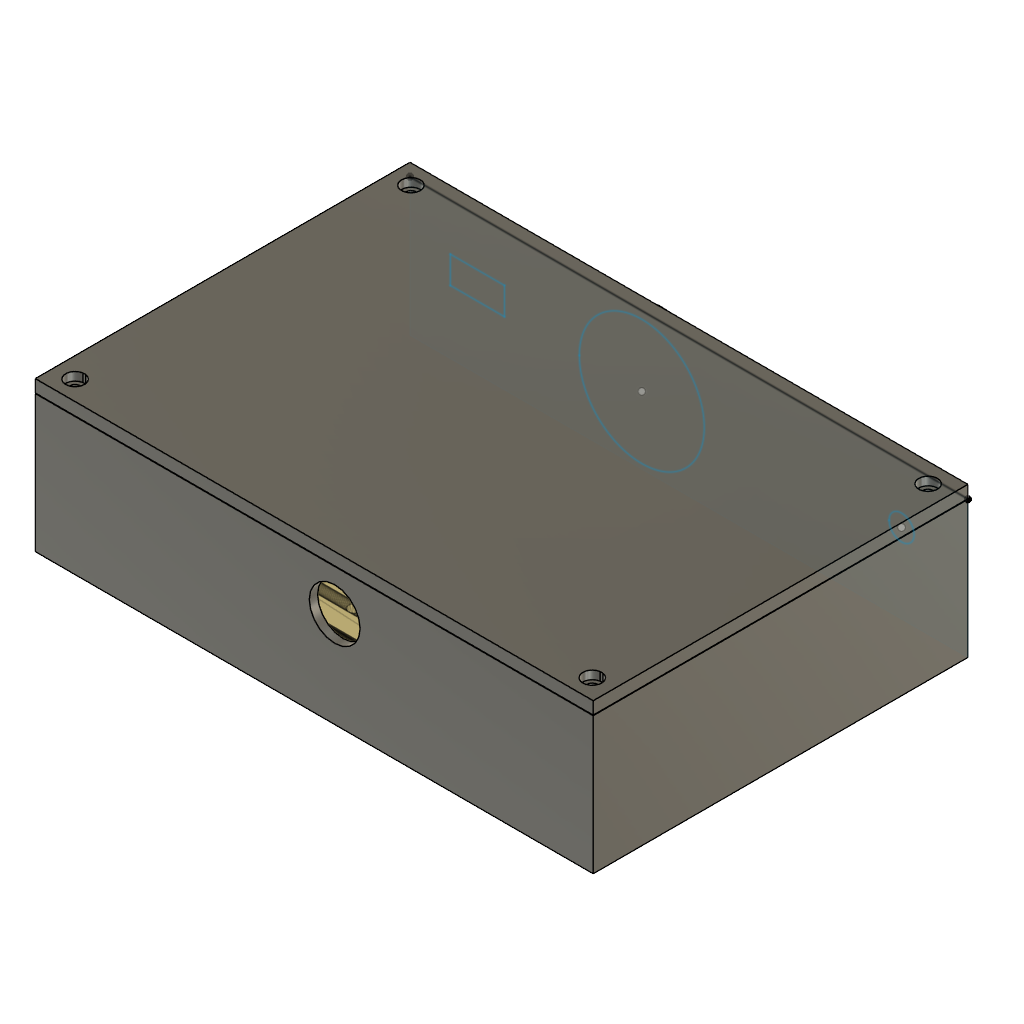
TerraVisionEnclosure (Autodesk Fusion 360 design; units mm, degrees)
part number: 2026-09-30-11-54-39-312
Autodesk Fusion 360 part; units mm, degrees
note: some values were not read from the file. Chosen so that the rebuilt part matches the saved one: which bodies a step acts on.
other "Elemento de malla base1"
other "Modificar1"
other "Modificar2"
other "Modificar3"
other "Modificar4"
other "Modificar5"
other "Modificar6"
other "Escala1"
other "Escala2"
other "Modificar7"
other "Modificar8"
other "Escala3"
sketch "Boceto3" plane through (0, 0, 0) normal (0, 0, 1) x (1, 0, 0)
  line L0 (-37.6392, 3.7951) -> (92.3608, 3.7951)
  line L1 (92.3608, 3.7951) -> (92.3608, 89.7951)
  line L2 (92.3608, 89.7951) -> (-37.6392, 89.7951)
  line L3 (-37.6392, 89.7951) -> (-37.6392, 3.7951)
  line L4 (92.1467, 91.7951) -> (-3.8533, 91.7951)
  line L5 (-3.8533, 1.7951) -> (92.1467, 1.7951)
  line L6 (94.3608, 1.7951) -> (94.3608, 91.7951)
  line L7 (94.3608, 91.7951) -> (-39.6392, 91.7951)
  line L8 (-39.6392, 91.7951) -> (-39.6392, 1.7951)
  line L9 (-39.6392, 1.7951) -> (94.3608, 1.7951)
  dimension "d25" = 130
  dimension "d26" = 86
  dimension "d27" = 2
  dimension "d28" = 2
  dimension "d29" = 2
  constraint horizontal L0
  constraint vertical L1
  constraint horizontal L2
  constraint vertical L3
  measures "d25" distance of L0.start L0.end
  measures "d26" distance of L0.end L1.end
extrude "Extruir1" add sketch "Boceto3" along normal blind 22 makes body 1
extrude "Extruir2" add 1 faces at (16.9561, 3.1284, 0) along direction (0, 0, -1) blind 2 on bodies 1 bodies 1
sketch "Boceto4" plane through (0, 0, -2) normal (0, 0, -1) x (1, 0, 0)
  line L0 (-37.6392, -89.7951) -> (-37.6392, -3.7951)
  line L1 (-37.6392, -3.7951) -> (92.3608, -3.7951)
  line L2 (92.3608, -3.7951) -> (92.3608, -89.7951)
  line L3 (92.3608, -89.7951) -> (-37.6392, -89.7951)
  line L4 (94.3608, -1.7951) -> (-39.6392, -1.7951)
  line L5 (-39.6392, -1.7951) -> (-39.6392, -91.7951)
  line L6 (-39.6392, -91.7951) -> (94.3608, -91.7951)
  line L7 (94.3608, -91.7951) -> (94.3608, -1.7951)
  line L8 (-39.6392, -1.7951) -> (94.3608, -1.7951)
  line L9 (94.3608, -1.7951) -> (94.3608, -91.7951)
  line L10 (94.3608, -91.7951) -> (-39.6392, -91.7951)
  line L11 (-39.6392, -91.7951) -> (-39.6392, -1.7951)
  line L12 (82.0002, -74) -> (87.2008, -74)
  line L13 (87.2008, -74) -> (87.2008, -77.8403)
  line L14 (87.2008, -77.8403) -> (82.0002, -77.8403)
  line L15 (82.0002, -77.8403) -> (82.0002, -74)
  line L16 (82.0002, -81.3917) -> (87.2008, -81.3917)
  line L17 (87.2008, -85.232) -> (82.0002, -85.232)
  line L18 (87.2008, -81.3917) -> (87.2008, -85.232)
  line L19 (82.0002, -85.232) -> (82.0002, -81.3917)
  line L20 (74.8756, -77.0003) -> (76.4831, -77.0003)
  line L21 (76.4831, -77.0003) -> (76.4831, -76.1982)
  line L22 (76.4831, -76.1982) -> (74.8756, -76.1982)
  line L23 (74.8756, -76.1982) -> (74.8756, -77.0003)
  line L24 (74.8706, -80.211) -> (76.4756, -80.211)
  line L25 (76.4756, -80.211) -> (76.4756, -81.0109)
  line L26 (76.4756, -81.0109) -> (74.8706, -81.0109)
  line L27 (74.8706, -81.0109) -> (74.8706, -80.211)
  line L28 (74.8675, -84.2259) -> (76.4935, -84.2259)
  line L29 (76.4935, -84.2259) -> (76.4935, -85.03)
  line L30 (76.4935, -85.03) -> (74.8675, -85.03)
  line L31 (74.8675, -85.03) -> (74.8675, -84.2259)
  line L32 (47.4882, -75.4522) -> (-31.5118, -75.4522)
  line L33 (-31.5118, -75.4522) -> (-31.5118, -37.9522)
  line L34 (-31.5118, -37.9522) -> (47.4882, -37.9522)
  line L35 (47.4882, -37.9522) -> (47.4882, -75.4522)
  circle A0 centre (77.0608, -61.7951) radius 6.5901
  line L36 (91.2608, -20.8951) -> (72.7608, -20.8951)
  line L37 (72.7608, -20.8951) -> (72.7608, -8.3951)
  line L38 (72.7608, -8.3951) -> (91.2608, -8.3951)
  line L39 (91.2608, -8.3951) -> (91.2608, -20.8951)
  circle A1 centre (51.0882, -73.0611) radius 2.25
  line L40 (7.9882, -33.9133) -> (7.9882, -79.4911) construction
  line L41 (51.6834, -56.7022) -> (-35.707, -56.7022) construction
  circle A2 centre (-35.1118, -73.0611) radius 2.25
  circle A3 centre (51.0882, -40.3432) radius 2.25
  circle A4 centre (-35.1118, -40.3432) radius 2.25
  circle A5 centre (3.5125, -87.4511) radius 1.5
  circle A6 centre (89.717, -87.3038) radius 1.5
  circle A7 centre (4.2711, -6.0742) radius 1.5
  circle A8 centre (89.46, -6.47) radius 1.5
  circle A9 centre (89.717, -87.3038) radius 1
  circle A10 centre (3.5125, -87.4511) radius 1
  circle A11 centre (4.2711, -6.0742) radius 1
  circle A12 centre (89.46, -6.47) radius 1
  point P0 (7.9882, -56.7022)
  point P1 (7.9882, -56.7022)
  dimension "d34" = 79
  dimension "d35" = 37.5
  dimension "d36" = 15.3
  dimension "d45" = 5.16
  dimension "d46" = 5.16
  dimension "d47" = 18.5
  dimension "d48" = 12.5
  dimension "d49" = 4.6
  dimension "d50" = 1.1
  dimension "d51" = 58
  dimension "d52" = 3.6
  dimension "d54" = 4.5
  dimension "d55" = 39.5
  dimension "d56" = 18.75
  dimension "d57" = 3
  dimension "d84" = -0.5
  dimension "d85" = -0.5
  dimension "d86" = -0.5
  dimension "d87" = -0.5
  constraint horizontal L8
  constraint vertical L9
  constraint horizontal L10
  constraint vertical L11
  constraint coincident L6.end L7.start
  constraint coincident L4.end L5.start
  constraint horizontal L12
  constraint vertical L13
  constraint horizontal L14
  constraint vertical L15
  constraint horizontal L16
  constraint vertical L18
  constraint horizontal L17
  constraint vertical L19
  constraint equal L12 L16
  constraint equal L15 L19
  constraint horizontal L20
  constraint vertical L21
  constraint horizontal L22
  constraint vertical L23
  constraint horizontal L24
  constraint vertical L25
  constraint horizontal L26
  constraint vertical L27
  constraint horizontal L28
  constraint vertical L29
  constraint horizontal L30
  constraint vertical L31
  constraint horizontal L32
  constraint vertical L33
  constraint horizontal L34
  constraint vertical L35
  constraint horizontal L36
  constraint vertical L37
  constraint horizontal L38
  constraint vertical L39
  constraint midpoint L40 P1
  constraint perpendicular L32 L40
  constraint midpoint L41 P1
  constraint coincident P1 P0
  constraint perpendicular L33 L41
  constraint symmetric A1 L40 A2
  constraint symmetric A1 L41 A3
  constraint symmetric L41 A2 A4
  constraint equal A5 A6
  constraint equal A5 A7
  constraint equal A5 A8
  measures "d34" distance of L32.start L32.end
  measures "d35" distance of L32.end L33.end
  measures "d36" distance of L2 A0.centre
  measures "d45" distance of L2 L13.end
  measures "d46" distance of L2 L17.start
  measures "d47" distance of L36.start L36.end
  measures "d48" distance of L36.start L38.end
  measures "d49" distance of L1 L38.end
  measures "d50" distance of L2 L38.end
  measures "d51" distance of L1 A0.centre
  measures "d52" distance of L35 A1.centre
  measures "d54" diameter of A1
  measures "d55" distance of L35 P1
  measures "d56" distance of L32 P1
  measures "d57" diameter of A5
extrude "Extruir6" add sketch "Boceto4" along normal blind 2 separate body contours L0 L1 L2 L3 makes body 2
extrude "Extruir7" add 1 faces at (49.0275, 2.4617, -2) along direction (0, 0, -1) blind 2 on bodies 1 bodies 1 2
extrude "Extruir8" add sketch "Boceto4" against normal blind 10 separate body contours A6 | A9 makes body 3
extrude "Extruir9" add sketch "Boceto4" against normal blind 10 separate body contours A5 | A7 | A8 | A10 | A11 | A12 makes body 4 at (4.9221, 86.9381, 4.6667) makes body 5 at (5.7693, 6.149, 4.6667) makes body 6 at (90.9581, 6.5448, 4.6667)
extrude "Extruir10" add 1 faces at (49.0275, 2.4617, 22) along direction (0, 0, 1) blind 7 on bodies 1 bodies 1
sketch "Boceto5" plane through (0, 1.7951, 0) normal (0, -1, 0) x (1, 0, 0)
  line L0 (94.3608, -4) -> (94.3608, 29)
  line L1 (94.3608, 29) -> (-39.6392, 29)
  line L2 (-39.6392, 29) -> (-39.6392, -4)
  line L3 (-39.6392, -4) -> (94.3608, -4)
  circle A0 centre (32.2847, 19) radius 6.1
  dimension "d68" = 12.2
  dimension "d69" = 33
  dimension "d70" = 23
  measures "d68" diameter of A0
  measures "d69" distance of L1 L3
  measures "d70" distance of L3 A0.centre
extrude "Extruir11" cut sketch "Boceto5" along normal blind -4 and the other way blind 0 contours A0 bodies 1
sketch "Boceto6" plane through (0, 91.7951, 0) normal (0, 1, 0) x (-1, 0, 0)
  line L0 (39.6392, -4) -> (39.6392, 29)
  line L1 (39.6392, 29) -> (-94.3608, 29)
  line L2 (-94.3608, 29) -> (-94.3608, -4)
  line L3 (-94.3608, -4) -> (39.6392, -4)
  line L4 (16.9478, 17.7095) -> (29.9478, 17.7095)
  line L5 (29.9478, 17.7095) -> (29.9478, 11.2095)
  line L6 (29.9478, 11.2095) -> (16.9478, 11.2095)
  line L7 (16.9478, 11.2095) -> (16.9478, 17.7095)
  circle A0 centre (-16.0339, 12.159) radius 15
  line L8 (39.6392, 29) -> (-94.3608, 29)
  line L9 (-94.3608, 29) -> (-94.3608, 28.9)
  line L10 (-94.3608, 28.9) -> (39.6392, 28.9)
  line L11 (39.6392, 28.9) -> (39.6392, 29)
  circle A1 centre (-78.4151, 15.0544) radius 3
  dimension "d75" = 6.5
  dimension "d76" = 13
  dimension "d77" = 30
  dimension "d135" = 0.1
  dimension "d141" = 6
  dimension "d146" = 33
  constraint horizontal L4
  constraint vertical L5
  constraint horizontal L6
  constraint vertical L7
  constraint horizontal L8
  constraint vertical L9
  constraint horizontal L10
  constraint vertical L11
  constraint coincident L2 L9.end
  constraint coincident L0.end L1.start
  measures "d75" distance of L4.end L5.end
  measures "d76" distance of L4.start L4.end
  measures "d77" diameter of A0
  measures "d135" distance of L0.end L10.end
  measures "d141" diameter of A1
  measures "d146" distance of L1.end L2.end
extrude "Extruir12" cut sketch "Boceto6" along normal blind -3 and the other way blind 0 contours L4 L5 L6 L7 bodies 1
extrude "Extruir13" add sketch "Boceto6" along normal blind 5 contours A0 bodies 1
extrude "Extruir14" cut sketch "Boceto4" against normal blind 10 contours A9 | A10 | A11 | A12 bodies 3 4 5 6
extrude "Extruir15" cut sketch "Boceto4" against normal blind 9 contours A5 | A6 | A7 | A8 bodies 3 4 5 6
sketch "Boceto7" plane through (0, 0, 29) normal (0, 0, 1) x (-1, 0, 0)
  line L0 (37.6392, -3.7951) -> (37.6392, -89.7951)
  line L1 (37.6392, -89.7951) -> (-92.3608, -89.7951)
  line L2 (-92.3608, -89.7951) -> (-92.3608, -3.7951)
  line L3 (-92.3608, -3.7951) -> (37.6392, -3.7951)
  line L4 (39.6392, -1.7951) -> (-94.3608, -1.7951)
  line L5 (-94.3608, -1.7951) -> (-94.3608, -91.7951)
  line L6 (-94.3608, -91.7951) -> (39.6392, -91.7951)
  line L7 (39.6392, -91.7951) -> (39.6392, -1.7951)
  line L8 (-89.1409, -8.6913) -> (-93.1409, -8.6913)
  line L9 (-93.1409, -8.6913) -> (-93.1409, -4.1913)
  line L10 (-93.1409, -4.1913) -> (-89.1409, -4.1913)
  line L11 (-87.1409, -6.1913) -> (-87.1409, -6.6913)
  arc A0 (-89.1409, -8.6913) -> (-87.1409, -6.6913) centre (-89.1409, -6.6913) ccw
  arc A1 (-87.1409, -6.1913) -> (-89.1409, -4.1913) centre (-89.1409, -6.1913) ccw
  circle A2 centre (-89.4569, -6.4674) radius 1.25
  line L12 (-94.3608, -1.7951) -> (-94.3608, -91.7951)
  line L13 (39.6392, -1.7951) -> (-94.3608, -1.7951)
  line L14 (65.6667, -46.7951) -> (-130, -46.7951) construction
  line L15 (-27.3608, -145) -> (-27.3608, 15) construction
  arc A3 (-87.1409, -86.8988) -> (-89.1409, -84.8988) centre (-89.1409, -86.8988) ccw
  line L16 (-89.1409, -84.8988) -> (-93.1409, -84.8988)
  line L17 (-93.1409, -84.8988) -> (-93.1409, -89.3988)
  line L18 (-93.1409, -89.3988) -> (-89.1409, -89.3988)
  arc A4 (-89.1409, -89.3988) -> (-87.1409, -87.3988) centre (-89.1409, -87.3988) ccw
  line L19 (-87.1409, -87.3988) -> (-87.1409, -86.8988)
  circle A5 centre (-89.4569, -87.1227) radius 1.25
  arc A6 (32.4192, -87.3988) -> (34.4192, -89.3988) centre (34.4192, -87.3988) ccw
  line L20 (38.4192, -89.3988) -> (34.4192, -89.3988)
  line L21 (38.4192, -84.8988) -> (38.4192, -89.3988)
  line L22 (34.4192, -84.8988) -> (38.4192, -84.8988)
  circle A7 centre (34.7353, -87.1227) radius 1.25
  arc A8 (34.4192, -84.8988) -> (32.4192, -86.8988) centre (34.4192, -86.8988) ccw
  line L23 (32.4192, -87.3988) -> (32.4192, -86.8988)
  line L24 (34.4192, -8.6913) -> (38.4192, -8.6913)
  line L25 (38.4192, -8.6913) -> (38.4192, -4.1913)
  line L26 (38.4192, -4.1913) -> (34.4192, -4.1913)
  arc A9 (34.4192, -4.1913) -> (32.4192, -6.1913) centre (34.4192, -6.1913) ccw
  arc A10 (32.4192, -6.6913) -> (34.4192, -8.6913) centre (34.4192, -6.6913) ccw
  line L27 (32.4192, -6.1913) -> (32.4192, -6.6913)
  circle A11 centre (34.7353, -6.4674) radius 1.25
  point P0 (-32.1667, -46.7951)
  point P1 (-27.3608, -65)
  dimension "d92" = 2
  dimension "d93" = 2
  dimension "d94" = 4.5
  dimension "d95" = 2.5
  dimension "d96" = 4
  dimension "d97" = 2
  dimension "d98" = 90
  dimension "d99" = 134
  dimension "d100" = 45
  dimension "d101" = 67
  constraint horizontal L8
  constraint vertical L9
  constraint horizontal L10
  constraint vertical L11
  constraint tangent L8 A0
  constraint tangent L11 A0
  constraint tangent L11 A1
  constraint tangent L10 A1
  constraint midpoint L14 P0
  constraint horizontal L14
  constraint midpoint L15 P1
  constraint perpendicular L13 L15
  constraint symmetric L8.end L14 L16.end
  constraint symmetric L9.end L14 L17.end
  constraint symmetric L8.start L14 A3.end
  constraint symmetric L11.end L14 A3.start
  constraint symmetric A0 L14 A3
  constraint symmetric L11.start L14 A4.end
  constraint symmetric L10.end L14 L18.end
  constraint symmetric A1 L14 A4
  constraint symmetric A2 L14 A5
  constraint symmetric L8.end L15 L24.end
  constraint symmetric L9.end L15 L25.end
  constraint symmetric L8.start L15 L24.start
  constraint symmetric L11.end L15 A10.start
  constraint symmetric A0 L15 A10
  constraint symmetric L11.start L15 A9.end
  constraint symmetric L10.end L15 L26.end
  constraint symmetric A1 L15 A9
  constraint symmetric A2 L15 A11
  constraint symmetric L15 A3.end L22.start
  constraint symmetric L15 A3.start A8.end
  constraint symmetric L15 A3 A8
  constraint symmetric L15 L16.end L21.start
  constraint symmetric L15 L17.end L20.start
  constraint symmetric L15 L18.end A6.end
  constraint symmetric L15 A4.end A6.start
  constraint symmetric L15 A4 A6
  constraint symmetric L15 A5 A7
  measures "d92" radius of A0
  measures "d93" radius of A1
  measures "d94" distance of L8.end L9.end
  measures "d95" diameter of A2
  measures "d96" distance of L8.end L8.start
  measures "d97" horizontal distance of L8.start L11.end
  measures "d98" distance of L4.end L5.end
  measures "d99" distance of L4.end L4.start
  measures "d100" distance of L13 L14
  measures "d101" distance of L12 L15
extrude "Extruir16" add sketch "Boceto7" against normal blind 2 contours L0 L24 L26 A9 A10 L27 | L2 L8 L10 L11 A0 A1 | L0 A6 L20 L22 A8 L23 | L2 A3 L16 L18 A4 L19 bodies 1
sketch "Boceto8" plane through (0, 0, 29) normal (0, 0, 1) x (-1, 0, 0)
  circle A0 centre (34.7353, -6.4674) radius 1.25
  circle A1 centre (34.7353, -87.1227) radius 1.25
  circle A2 centre (-89.4569, -6.4674) radius 1.25
  circle A3 centre (-89.4569, -87.1227) radius 1.25
  line L0 (37.6392, -3.7951) -> (37.6392, -4.1913)
  line L1 (37.6392, -4.1913) -> (34.4192, -4.1913)
  arc A4 (34.4192, -4.1913) -> (32.4192, -6.1913) centre (34.4192, -6.1913) ccw
  line L2 (32.4192, -6.1913) -> (32.4192, -6.6913)
  arc A5 (32.4192, -6.6913) -> (34.4192, -8.6913) centre (34.4192, -6.6913) ccw
  line L3 (34.4192, -8.6913) -> (37.6392, -8.6913)
  line L4 (37.6392, -8.6913) -> (37.6392, -84.8988)
  line L5 (37.6392, -84.8988) -> (34.4192, -84.8988)
  arc A6 (34.4192, -84.8988) -> (32.4192, -86.8988) centre (34.4192, -86.8988) ccw
  line L6 (32.4192, -86.8988) -> (32.4192, -87.3988)
  arc A7 (32.4192, -87.3988) -> (34.4192, -89.3988) centre (34.4192, -87.3988) ccw
  line L7 (34.4192, -89.3988) -> (37.6392, -89.3988)
  line L8 (37.6392, -89.3988) -> (37.6392, -89.7951)
  line L9 (37.6392, -89.7951) -> (-92.3608, -89.7951)
  line L10 (-92.3608, -89.7951) -> (-92.3608, -89.3988)
  line L11 (-92.3608, -89.3988) -> (-89.1409, -89.3988)
  arc A8 (-89.1409, -89.3988) -> (-87.1409, -87.3988) centre (-89.1409, -87.3988) ccw
  line L12 (-87.1409, -87.3988) -> (-87.1409, -86.8988)
  arc A9 (-87.1409, -86.8988) -> (-89.1409, -84.8988) centre (-89.1409, -86.8988) ccw
  line L13 (-89.1409, -84.8988) -> (-92.3608, -84.8988)
  line L14 (-92.3608, -84.8988) -> (-92.3608, -8.6913)
  line L15 (-92.3608, -8.6913) -> (-89.1409, -8.6913)
  arc A10 (-89.1409, -8.6913) -> (-87.1409, -6.6913) centre (-89.1409, -6.6913) ccw
  line L16 (-87.1409, -6.6913) -> (-87.1409, -6.1913)
  arc A11 (-87.1409, -6.1913) -> (-89.1409, -4.1913) centre (-89.1409, -6.1913) ccw
  line L17 (-89.1409, -4.1913) -> (-92.3608, -4.1913)
  line L18 (-92.3608, -4.1913) -> (-92.3608, -3.7951)
  line L19 (-92.3608, -3.7951) -> (37.6392, -3.7951)
  line L20 (39.6392, -1.7951) -> (-94.3608, -1.7951)
  line L21 (-94.3608, -1.7951) -> (-94.3608, -91.7951)
  line L22 (-94.3608, -91.7951) -> (39.6392, -91.7951)
  line L23 (39.6392, -91.7951) -> (39.6392, -1.7951)
  line L24 (39.6392, -1.7951) -> (-94.3608, -1.7951)
  line L25 (-94.3608, -1.7951) -> (-94.3608, -91.7951)
  line L26 (-94.3608, -91.7951) -> (39.6392, -91.7951)
  line L27 (39.6392, -91.7951) -> (39.6392, -1.7951)
  circle A12 centre (34.7353, -87.1227) radius 1.25
  circle A13 centre (-89.4569, -87.1227) radius 1.25
  circle A14 centre (-89.4569, -6.4674) radius 1.25
  circle A15 centre (34.7353, -6.4674) radius 1.25
  circle A16 centre (34.7353, -87.1227) radius 2.25
  circle A17 centre (-89.4569, -87.1227) radius 2.25
  circle A18 centre (-89.4569, -6.4674) radius 2.25
  circle A19 centre (34.7353, -6.4674) radius 2.25
  dimension "d104" = 134
  dimension "d105" = 90
  dimension "d108" = 1
  dimension "d109" = 1
  dimension "d110" = 1
  dimension "d111" = 1
  constraint horizontal L24
  constraint vertical L25
  constraint horizontal L26
  constraint vertical L27
  constraint coincident L21.end L22.start
  constraint coincident L20.start L23.end
  constraint concentric A1 A12
  constraint concentric A3 A13
  constraint concentric A2 A14
  constraint concentric A0 A15
  measures "d104" distance of L21.end L22.end
  measures "d105" distance of L20.end L21.end
extrude "Extruir17" add sketch "Boceto8" along normal blind 3 contours L0 L1 A4 L2 A5 L3 L4 L5 A6 L6 A7 L7 L8 L9 L10 L11 A8 L12 A9 L13 L14 L15 A10 L16 A11 L17 L18 L19 A16 A17 A18 A19 | A5 L3 A19 | A5 L3 A19 | L15 A10 A18 | L15 A10 A18 | L5 A6 A16 | L5 A6 A16 | A9 L13 A17 | A9 L13 A17 | L20 L21 L22 L23 L24 L25 L26 L27 bodies 1
extrude "Extruir18" cut sketch "Boceto8" along normal blind 2 from surface at -1 contours A5 L3 A19 | L15 A10 A18 | L5 A6 A16 | A9 L13 A17 picked at (34.7749, -8.3655) picked at (-89.4965, -8.3655) picked at (34.7749, -85.2246) picked at (-89.4965, -85.2246) bodies 1
extrude "Extruir19" cut sketch "Boceto8" along normal blind 2 from surface at 1 contours L15 A10 A18 picked at (-89.4965, -8.3655) bodies 1
extrude "Extruir20" cut sketch "Boceto8" along normal blind 2 from surface at 1 contours A9 L13 A17 picked at (-89.4965, -85.2246) bodies 1
extrude "Extruir21" cut sketch "Boceto8" along normal blind 2 from surface at 1 contours A5 L3 A19 picked at (34.7749, -8.3655) bodies 1
extrude "Extruir22" cut sketch "Boceto8" along normal blind 2 from surface at 1 contours L5 A6 A16 picked at (34.7749, -85.2246) bodies 1
extrude "Extruir23" add sketch "Boceto8" along normal blind 1 contours L5 A6 A16 picked at (34.7749, -85.2246) bodies 1
extrude "Extruir24" add sketch "Boceto8" along normal blind 1 contours A9 L13 A17 picked at (-89.4965, -85.2246) bodies 1
extrude "Extruir25" add sketch "Boceto8" along normal blind 1 contours L15 A10 A18 picked at (-89.4965, -8.3655) bodies 1
extrude "Extruir26" add sketch "Boceto8" along normal blind 1 contours A5 L3 A19 picked at (34.7749, -8.3655) bodies 1
extrude "Extruir27" cut sketch "Boceto6" along normal through all and the other way through all contours L0 L1 L2 L8 L9 L10 L11 bodies 1 makes body 7 at (47.6664, 33.5974, 29)
sketch "Boceto9" plane through (0, 96.7951, 0) normal (0, 1, 0) x (-1, 0, 0)
  circle A0 centre (-16.0339, 12.159) radius 15
  circle A1 centre (-7.4096, 20.674) radius 2
  line L0 (-16.0339, 39.9175) -> (-16.0339, -15.5995) construction
  line L1 (-37.1309, 12.159) -> (5.0632, 12.159) construction
  circle A2 centre (-7.4096, 3.644) radius 2
  circle A3 centre (-24.6581, 20.674) radius 2
  circle A4 centre (-24.6581, 3.644) radius 2
  point P0 (-16.0339, 12.159)
  point P1 (-16.0339, 12.159)
  point P2 (-16.0339, 12.159)
  point P3 (-16.0339, 12.159)
  point P4 (-16.0339, 12.159)
  dimension "d138" = 4
  constraint coincident P4 P2
  constraint coincident P3 P2
  constraint midpoint L0 P4
  constraint vertical L0
  constraint coincident P4 P3
  constraint midpoint L1 P4
  constraint perpendicular L0 L1
  constraint symmetric A1 L1 A2
  constraint symmetric A1 L0 A3
  constraint symmetric L0 A2 A4
  measures "d138" diameter of A1
extrude "Extruir28" cut sketch "Boceto9" against normal blind 5 contours A1 | A2 | A3 | A4 bodies 1
extrude "Extruir29" cut sketch "Boceto6" along normal blind 2 and the other way blind 2 contours A1 bodies 1
extrude "Extruir3" [suppressed]
extrude "Extruir4" [suppressed]
extrude "Extruir5" [suppressed]
